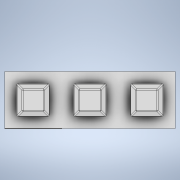
# Autodesk Inventor part: 1x3 button cover
Saved by Autodesk Inventor 2022 (Build 260153000, 153)
## iProperties
Created: 2022-05-03
Part Number: 1x3 button cover
Material: Generic
Document SubType Name: Modeling
Designer: a-dubs
Density: 1 g/cm^3
Appearance: Default
Author: a-dubs
Autodesk Inventor part; units mm, degrees
ref_plane "YZ Plane" through (0, 0, 0) normal (1, 0, 0) x (0, 1, 0)
ref_plane "XZ Plane" through (0, 0, 0) normal (0, 1, 0) x (-1, 0, 0)
ref_plane "XY Plane" through (0, 0, 0) normal (0, 0, 1) x (1, 0, 0)
sketch "Sketch1" plane through (0, 0, 0) normal (0, 1, 0) x (-1, 0, 0)
  line L0 (2.95, 2.95) -> (-2.95, 2.95)
  line L1 (-2.95, 2.95) -> (-2.95, -2.95)
  line L2 (-2.95, -2.95) -> (2.95, -2.95)
  line L3 (2.95, -2.95) -> (2.95, 2.95)
  line L4 (2.95, 2.95) -> (-2.95, -2.95) construction
  line L5 (-2.95, 2.95) -> (2.95, -2.95) construction
  line L6 (-2.95, -2.95) -> (-2.95, -7.504)
  line L7 (-2.95, -7.504) -> (-7.504, -7.504)
  line L8 (7.504, 7.504) -> (-7.504, 7.504)
  line L9 (-7.504, 7.504) -> (-7.504, -7.504)
  line L10 (-7.504, -7.504) -> (7.504, -7.504)
  line L11 (7.504, -7.504) -> (7.504, 7.504)
  line L12 (7.504, 7.504) -> (-7.504, -7.504) construction
  line L13 (-7.504, 7.504) -> (7.504, -7.504) construction
  circle A0 centre (0, 0) radius 1.7
  line L14 (2.95, 2.95) -> (1.2021, 1.2021)
  circle A1 centre (2.076, 2.076) radius 0.5
  line L15 (0, 0) -> (0, 1)
  circle A2 centre (-2.076, 2.076) radius 0.5
  line L16 (0, 0) -> (-0.5185, 0)
  circle A3 centre (2.076, -2.076) radius 0.5
  circle A4 centre (-2.076, -2.076) radius 0.5
  line L17 (2.95, -2.95) -> (2.95, -2.7)
  line L18 (2.95, -2.7) -> (3.25, -2.7)
  line L19 (3.25, -2.7) -> (3.25, -1.95)
  line L20 (3.25, -1.95) -> (2.95, -1.95)
  line L21 (2.95, -1.95) -> (2.95, -2.7)
  line L22 (-2.95, -2.95) -> (2.95, 2.95) construction
  line L23 (2.95, 2.7) -> (3.25, 2.7)
  line L24 (3.25, 2.7) -> (3.25, 1.95)
  line L25 (3.25, 1.95) -> (2.95, 1.95)
  line L26 (2.95, 1.95) -> (2.95, 2.7)
  line L27 (-2.95, -2.7) -> (-3.25, -2.7)
  line L28 (-3.25, -2.7) -> (-3.25, -1.95)
  line L29 (-3.25, -1.95) -> (-2.95, -1.95)
  line L30 (-3.25, 1.95) -> (-2.95, 1.95)
  line L31 (-2.95, 2.7) -> (-3.25, 2.7)
  line L32 (-3.25, 2.7) -> (-3.25, 1.95)
  line L33 (-2.95, -2.95) -> (-2.95, -4.35)
  line L34 (-2.95, -4.35) -> (-4.35, -4.35)
  line L35 (4.35, 4.35) -> (-4.35, 4.35)
  line L36 (-4.35, 4.35) -> (-4.35, -4.35)
  line L37 (-4.35, -4.35) -> (4.35, -4.35)
  line L38 (4.35, -4.35) -> (4.35, 4.35)
  line L39 (4.35, 4.35) -> (-4.35, -4.35) construction
  line L40 (-4.35, 4.35) -> (4.35, -4.35) construction
  circle A5 centre (0, 0) radius 2.2
  line L41 (2.95, 1.1907) -> (1.1907, 2.95)
  line L42 (-1.1907, 2.95) -> (-2.95, 1.1907)
  line L43 (-2.95, -1.1907) -> (-1.1907, -2.95)
  line L44 (1.1907, -2.95) -> (2.95, -1.1907)
  line L45 (3.35, -3.35) -> (-3.35, -3.35)
  line L46 (-3.35, -3.35) -> (-3.35, 3.35)
  line L47 (-3.35, 3.35) -> (3.35, 3.35)
  line L48 (3.35, 3.35) -> (3.35, -3.35)
  line L49 (3.35, -3.35) -> (-3.35, 3.35) construction
  line L50 (-3.35, -3.35) -> (3.35, 3.35) construction
  line L51 (-2.95, 2.95) -> (-3.35, 2.95)
  line L52 (-2.95, -2.95) -> (-2.95, -3.35)
  line L53 (-3.35, -2.95) -> (-4.35, -2.95)
  line L54 (-2.95, 3.35) -> (-2.95, 4.35)
  point P0 (-2.95, 1.1907)
  dimension "d12" = 3.4
  dimension "d6" = 5.9
  dimension "d7" = 5.9
  dimension "d9" = 4.554
  dimension "d15" = 1
  dimension "d27" = 0.25
  dimension "d28" = 0.3
  dimension "d29" = 0.75
  dimension "d61" = 4.4
  dimension "d64" = 360
  dimension "d112" = 0.4
  dimension "d113" = 1
  dimension "d114" = 1
  constraints: 110 end point, 15 symmetric about line, 13 point on line, 11 perpendicular, 10 parallel, 9 midpoint, 7 horizontal, 5 centre point, 2 coincident, 2 vertical, 19 other
  measures "d6" distance of L0.start L0.end
  measures "d7" distance of L1.end L0.end
  measures "d9" distance of L6.end L7.end
  measures "d15" diameter of A1
  measures "d27" distance of L2.end L17.end
  measures "d28" distance of L20.end L19.end
  measures "d29" distance of L19.end L18.end
  measures "d61" diameter of A5
  measures "d112" distance of L0.end L51.end
  measures "d113" distance of L53.start L53.end
  measures "d114" distance of L54.start L54.end
extrude "Extrusion8" add sketch "Sketch1" along normal blind 4 contours L46 L53 L36 L35 L54 L47 | L46 L45 L6 L34 L36 L53 | L54 L35 L38 L37 L6 L45 L48 L47
extrude "Extrusion12" add sketch "Sketch1" along normal blind 1.5 from surface at 4 contours L14 A1 L41 L0 | L0 L51 L46 L47 L48 L45 L6 L2 L3 L18 L19 L20 L25 L24 L23 | L3 L41 A1 L14 | L41 A1 L3 L44 A3 L2 L43 A4 L1 L42 A2 L0 | L23 L24 L25 L3 | A1 L41 L14 | L14 L41 A1 | L42 A2 L1 L0 | L41 L14 A1 | L41 A1 L14 | L1 L31 L32 L30 L29 L28 L27 L6 L45 L46 L51 | L42 A2 | A2 L42 | L1 L30 L32 L31 | L46 L53 L36 L35 L54 L47 | L3 L2 L44 A3 | L46 L45 L6 L34 L36 L53 | L20 L19 L18 L3 | L44 A3 | A3 L44 | L54 L35 L38 L37 L6 L45 L48 L47 | L43 A4 L2 L1 | L1 L27 L28 L29 | L43 A4 | A4 L43 | A0 | A5
chamfer "Chamfer1" distance 0.5 angle 45 4 edges at (0, 4, 3.35) (-3.35, 4, 0) (0, 4, -3.35) (3.35, 4, 0)
chamfer "Chamfer2" distance 1.5 angle 45 4 edges at (0, 5.5, 4.35) (4.35, 5.5, 0) (0, 5.5, -4.35) (-4.35, 5.5, 0)
extrude "Extrusion13" add sketch "Sketch1" along normal blind 1 contours L7 L9 L8 L11 L10
fillet "Fillet8" radius 0.5 16 edges at (3.6, 4.75, -3.6) (0, 5.5, -2.85) (-3.6, 4.75, -3.6) (2.85, 5.5, 0) (3.6, 4.75, 3.6) (4.35, 4, 0) (0, 5.5, 2.85) (-3.6, 4.75, 3.6) (-2.85, 5.5, 0) (-4.35, 4, 0) (0, 4, 4.35) (-4.35, 2.5, 4.35) (-4.35, 2.5, -4.35) (0, 4, -4.35) (4.35, 2.5, -4.35) (4.35, 2.5, 4.35)
pattern_linear "Rectangular Pattern3" count 3 spacing 15.008 along (1, 0, 0) of "Extrusion8", "Extrusion12", "Chamfer1", "Chamfer2", "Extrusion13", "Fillet8"
body "Solid2"
